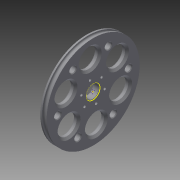
# Autodesk Inventor part: 7.25in Pully
Saved by Autodesk Inventor 2014 SP1 (Build 180222100, 222)
## iProperties
Created: 2014-01-29
Part Number: 7.25in Pully
Material: Generic
Document SubType Name: Modeling
Designer: Pradhan Alexander
Density: 1 g/cm^3
Appearance: Default
Author: Pradhan Alexander
Autodesk Inventor part; units mm, degrees
ref_plane "YZ Plane" through (0, 0, 0) normal (1, 0, 0) x (0, 1, 0)
ref_plane "XZ Plane" through (0, 0, 0) normal (0, 1, 0) x (-1, 0, 0)
ref_plane "XY Plane" through (0, 0, 0) normal (0, 0, 1) x (1, 0, 0)
sketch "Sketch1" plane through (0, 0, 0) normal (0, 0, 1) x (1, 0, 0)
  line L0 (-10.0445, -59.5143) -> (2.6555, -59.5143)
  line L1 (2.6555, -59.5143) -> (2.6555, 32.5607)
  line L2 (-10.0445, -59.5143) -> (-10.0445, 32.5607)
  line L3 (2.6555, 32.5607) -> (-0.5195, 32.5607)
  line L4 (-6.8695, 32.5607) -> (-10.0445, 32.5607)
  line L5 (-6.8695, 32.5607) -> (-6.8695, 32.1797)
  line L6 (-0.5195, 32.5607) -> (-0.5195, 32.1797)
  arc A0 (-6.8695, 32.1797) -> (-0.5195, 32.1797) centre (-3.6945, 32.1797) ccw
  point P0 (-8.457, 32.5607)
  point P1 (1.068, 32.5607)
  dimension "d0" = 12.7
  dimension "d3" = 92.075
  dimension "d4" = 0.381
  constraints: 14 end point, 3 equal length, 3 perpendicular, 2 midpoint, 2 point on circle, 2 tangent, 1 centre point, 1 horizontal, 1 horizontal alignment, 1 parallel
  measures "d0" distance between parallel lines of L1 L2
  measures "d3" distance of L0.start L2.end
  measures "d4" distance of L4.start L5.end
revolve "Revolution1" add sketch "Sketch1" angle 360 about axis through (-10.0445, -59.5143, 0) along (1, 0, 0)
sketch "Sketch2" plane through (2.6555, -59.5143, 0) normal (1, 0, 0) x (0, 0, -1)
  circle A0 centre (0, 0) radius 92.075 projected
  circle A1 centre (0, 0) radius 12.7
  dimension "d6" = 25.4
  constraints: 1 centre point, 1 coincident
  measures "d6" diameter of A1
extrude "Extrusion1" cut sketch "Sketch2" against normal blind 25.4 contours A1
sketch "Sketch3" plane through (1.7665, -59.5143, 0) normal (1, 0, 0) x (0, 0, -1)
  circle A0 centre (0, 0) radius 14.1224 projected
  constraints: 1 coincident
sketch "Sketch4" plane through (2.6555, -59.5143, 0) normal (1, 0, 0) x (0, 0, -1)
  circle A0 centre (16.847, 16.847) radius 2.54
  circle A1 centre (0, 0) radius 4.7625 projected
  line L0 (0, 0) -> (16.847, 16.847)
  dimension "d18" = 23.8252
  dimension "d24" = 5.08
  constraints: 2 end point, 1 centre point
  measures "d18" distance of L0.start L0.end
  measures "d24" diameter of A0
extrude "Extrusion2" cut sketch "Sketch4" against normal blind 10160 contours A0
pattern_circular "Circular Pattern1" count 6 over 360 about axis through (-258.9705, -59.5143, 0) along (1, 0, 0) of "Extrusion2"
sketch "Sketch5" plane through (2.6555, -59.5143, 0) normal (1, 0, 0) x (0, 0, -1)
  circle A0 centre (0, 0) radius 12.7 projected
  circle A1 centre (-6.1664, 58.928) radius 19.05
  dimension "d25" = 38.1
  dimension "d26" = 58.928
  constraints: 1 centre point
  measures "d25" diameter of A1
  measures "d26" vertical distance of A0.centre A1.centre
extrude "Extrusion3" cut sketch "Sketch5" against normal blind 25.4 contours A1
pattern_circular "Circular Pattern2" count 6 over 360 about axis through (2.6555, -59.5143, 0) along (-1, 0, 0) of "Extrusion3"
sketch "Sketch6" plane through (2.6555, -59.5143, 0) normal (1, 0, 0) x (0, 0, -1)
  circle A0 centre (0, 0) radius 12.7 projected
  circle A1 centre (0, 0) radius 92.075 projected
  circle A2 centre (0, 0) radius 14.224
  dimension "d32" = 28.448
  constraints: 1 centre point, 1 coincident
  measures "d32" diameter of A2
extrude "Extrusion4" cut sketch "Sketch6" against normal blind 0.889 contours A2
chamfer "Chamfer1" distance 3.81 angle 45 12 edges at (2.6555, -0.5863, 25.2164) (-10.0445, -0.5863, 25.2164) (2.6555, -8.2122, -38.4249) (-10.0445, -8.2122, -38.4249) (2.6555, -67.1402, -63.6414) (-10.0445, -67.1402, -63.6414) (2.6555, -118.4423, -25.2164) (-10.0445, -118.4423, -25.2164) (2.6555, -110.8163, 38.4249) (-10.0445, -110.8163, 38.4249) (2.6555, -51.8883, 63.6414) (-10.0445, -51.8883, 63.6414)
sketch "Sketch7" plane through (2.6555, -59.5143, 0) normal (1, 0, 0) x (0, 0, -1)
  circle A0 centre (-6.1664, 58.928) radius 22.86 projected
  circle A1 centre (-54.1164, 24.1237) radius 22.86 projected
  circle A2 centre (-39.8214, 57.7787) radius 6.35
  dimension "d38" = 12.7
  dimension "d39" = 33.655
  dimension "d40" = 33.655
  constraints: 1 centre point
  measures "d38" diameter of A2
  measures "d39" horizontal distance of A0.centre A2.centre
  measures "d40" vertical distance of A1.centre A2.centre
extrude "Extrusion5" cut sketch "Sketch7" against normal blind 50.8 contours A2
pattern_circular "Circular Pattern3" count 6 over 360 about axis through (2.6555, -59.5143, 0) along (-1, 0, 0) of "Extrusion5"
chamfer "Chamfer2" distance 1.27 angle 45 12 edges at (2.6555, -1.7355, 46.1714) (-10.0445, -1.7355, 46.1714) (2.6555, 9.3607, -26.9521) (-10.0445, 9.3607, -26.9521) (2.6555, -48.418, -73.1236) (-10.0445, -48.418, -73.1236) (2.6555, -117.293, -46.1714) (-10.0445, -117.293, -46.1714) (2.6555, -128.3893, 26.9521) (-10.0445, -128.3893, 26.9521) (-10.0445, -70.6105, 73.1236) (2.6555, -70.6105, 73.1236)
body "Solid1"
